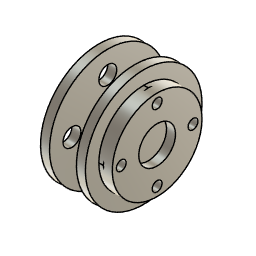
motor_shaft v5 (Autodesk Fusion 360 design; units mm, degrees)
Autodesk Fusion 360 part; units mm, degrees
note: some values were not read from the file. Set by a fixed rule: which sketch regions a step uses.
sketch "Sketch1" plane through (0, 0, 0) normal (0, 1, 0) x (1, 0, 0)
  line L0 (0, 0) -> (0, -10)
  line L1 (0, -10) -> (-2, -10)
  line L2 (-3, -13) -> (-5, -13)
  line L3 (-5, -13) -> (-5, -3)
  line L4 (-5, -3) -> (-11, -3)
  line L5 (-11, -3) -> (-11, -13)
  line L6 (-11, -13) -> (-13, -13)
  line L7 (-13, -13) -> (-13, 0)
  line L8 (-13, 0) -> (0, 0)
  line L9 (0, 0) -> (0, -4.1)
  line L10 (0, -4.1) -> (-2, -4.1)
  line L11 (-2, -4.1) -> (-2, 0)
  line L12 (-2, -10) -> (-3, -10)
  line L13 (-3, -10) -> (-3, -13)
  dimension "d1" = 10
  dimension "d2" = 2
  dimension "d3" = 4.1
  dimension "d17" = 1
  dimension "d18" = 2
  dimension "d19" = 6
  dimension "d20" = 2
  dimension "d21" = 13
  dimension "d24" = 3
  dimension "d25" = 3
  dimension "d26" = 13
  constraint coincident L0.start L8.end
  constraint vertical L0
  constraint perpendicular L0 L1
  constraint perpendicular L2 L3
  constraint perpendicular L3 L4
  constraint perpendicular L4 L5
  constraint perpendicular L5 L6
  constraint perpendicular L4 L7
  constraint perpendicular L0 L8
  constraint perpendicular L8 L9
  constraint perpendicular L9 L10
  constraint coincident L8 L11.end
  constraint perpendicular L8 L11
  constraint parallel L1 L12
  constraint perpendicular L2 L13
  measures "d1" distance of L0.start L0.end
  measures "d2" distance of L0.end L1.end
  measures "d3" distance of L0.start L9.end
  measures "d17" distance of L1.end L12.end
  measures "d18" distance of L2.start L2.end
  measures "d19" distance of L3.end L4.end
  measures "d20" distance of L5.end L6.end
  measures "d21" distance of L7.end L0.start
  measures "d24" distance of L4 L8
  measures "d25" distance of L2.start L12.end
  measures "d26" distance of L6.end L7.end
revolve "Revolve1" add sketch "Sketch1" angle 360 about axis through (1.75, 0, 0) along (1, 0, 0) contours L0 L1 L2 L3 L4 L5 L6 L7 L8 L10 L11 L12 L13
sketch "Sketch2" plane through (0, 0, 0) normal (1, 0, 0) x (0, 1, 0)
  circle A0 centre (0, 0) radius 4.1
  circle A1 centre (0, 0) radius 10
  circle A2 centre (0, 0) radius 8
  circle A3 centre (0, 8) radius 1.1
  circle A4 centre (-8, 0) radius 1.1
  circle A5 centre (8, 0) radius 1.1
  circle A6 centre (0, -8) radius 1.1
  dimension "d5" = 16
  dimension "d6" = 2.2
  dimension "d7" = 2.2
  dimension "d8" = 2.2
  dimension "d9" = 2.2
  constraint concentric A0 A2
  constraint coincident A2 A3.centre
  constraint coincident A2 A4.centre
  constraint coincident A2 A5.centre
  constraint coincident A2 A6.centre
  measures "d5" diameter of A2
  measures "d6" diameter of A3
  measures "d7" diameter of A4
  measures "d8" diameter of A5
  measures "d9" diameter of A6
extrude "Extrude1" cut sketch "Sketch2" against normal blind 20 contours A2 A5 | A2 A5 | A2 A3 | A2 A3 | A2 A6 | A2 A6 | A2 A4 | A2 A4
sketch "Sketch3" plane through (-13, 0, 0) normal (-1, 0, 0) x (0, -1, 0)
  circle A0 centre (8, 0) radius 1.1
  circle A1 centre (-8, 0) radius 1.1
  circle A2 centre (0, 8) radius 1.1
  circle A3 centre (0, -8) radius 1.1
  circle A4 centre (0, 0) radius 13
  circle A5 centre (0, 8) radius 2
  circle A6 centre (8, 0) radius 2
  circle A7 centre (0, -8) radius 2
  circle A8 centre (-8, 0) radius 2
  constraint concentric A2 A5
  constraint concentric A0 A6
  constraint concentric A3 A7
  constraint concentric A1 A8
extrude "Extrude2" cut sketch "Sketch3" against normal blind 11 contours A5 | A6 | A7 | A8
sketch "Sketch4" plane through (0, 0, 0) normal (0, 1, 0) x (1, 0, 0)
  circle A0 centre (-8, 0) radius 1
  line L0 (-5, 13) -> (-5, -13)
  dimension "d14" = 2
  dimension "d22" = 3
  measures "d14" diameter of A0
  measures "d22" distance of A0.centre L0
extrude "Extrude3" cut sketch "Sketch4" along normal through all and the other way through all
equation "d3 = ( 8.2 / 2 ) * 1 mm"
